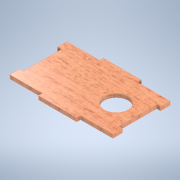
# Autodesk Inventor part: SideFemale_100wx60h
Saved by Autodesk Inventor 2022.2 (Build 262287000, 287)
## iProperties
Created: 2023-04-17
Part Number: SideFemale_100wx60h
Material: Wood (Oak)
Document SubType Name: Modeling
Designer: jaege
Density: 0.76 g/cm^3
Appearance: Red Oak - Natural Low Gloss
Author: jaege
Autodesk Inventor part; units mm, degrees
ref_plane "YZ Plane" through (0, 0, 0) normal (1, 0, 0) x (0, 1, 0)
ref_plane "XZ Plane" through (0, 0, 0) normal (0, 1, 0) x (-1, 0, 0)
ref_plane "XY Plane" through (0, 0, 0) normal (0, 0, 1) x (1, 0, 0)
sketch "Sketch1" plane through (0, 0, 0) normal (0, 1, 0) x (-1, 0, 0)
  line L0 (50, 30) -> (-50, 30) construction
  line L1 (-50, 30) -> (-50, -30) construction
  line L2 (-50, -30) -> (50, -30) construction
  line L3 (50, -30) -> (50, 30) construction
  line L4 (-50, -20) -> (-54, -20)
  line L5 (-54, -20) -> (-54, -30)
  line L6 (-54, -30) -> (-50, -30)
  line L7 (-50, -30) -> (-50, -20) construction
  line L8 (-50, 20) -> (-54, 20)
  line L9 (-54, 20) -> (-54, 30)
  line L10 (-54, 30) -> (-50, 30)
  line L11 (-50, 30) -> (-50, 20) construction
  line L12 (50, 30) -> (54, 30)
  line L13 (54, 30) -> (54, 20)
  line L14 (54, 20) -> (50, 20)
  line L15 (50, 20) -> (50, 30) construction
  line L16 (50, -30) -> (54, -30)
  line L17 (54, -30) -> (54, -20)
  line L18 (54, -20) -> (50, -20)
  line L19 (50, -20) -> (50, -30) construction
  line L20 (20, -30) -> (50, -30) construction
  line L21 (50, -30) -> (50, -34) construction
  line L22 (50, -34) -> (20, -34) construction
  line L23 (20, -34) -> (20, -30)
  line L24 (-20, -30) -> (-50, -30) construction
  line L25 (-50, -30) -> (-50, -34) construction
  line L26 (-50, -34) -> (-20, -34) construction
  line L27 (-20, -34) -> (-20, -30)
  line L28 (-50, 30) -> (-20, 30)
  line L29 (-20, 30) -> (-20, 34)
  line L30 (-20, 34) -> (-50, 34) construction
  line L31 (-50, 34) -> (-50, 30) construction
  line L32 (20, 34) -> (50, 34) construction
  line L33 (50, 34) -> (50, 30) construction
  line L34 (50, 30) -> (20, 30)
  line L35 (20, 30) -> (20, 34)
  line L36 (20, -30) -> (-20, -30) construction
  line L37 (-50, 20) -> (-50, -20)
  line L38 (50, -20) -> (50, 20)
  line L39 (20, 30) -> (-20, 30) construction
  line L40 (50, -30) -> (20, -30)
  line L41 (20, -34) -> (-20, -34)
  line L42 (-20, -30) -> (-50, -30)
  line L43 (-20, 34) -> (20, 34)
  line L44 (20, 30) -> (50, 30)
  point P0 (0, 0)
  point P1 (52, 20)
  point P2 (52, -20)
  point P3 (-20, -32)
  point P4 (20, -32)
  point P5 (0, -30)
  point P6 (50, 0)
  dimension "d0" = 100
  dimension "d1" = 60
  dimension "d2" = 4
  dimension "d3" = 40
  dimension "d4" = 40
  constraints: 90 end point, 20 parallel, 16 point on line, 12 perpendicular, 10 horizontal, 7 collinear, 6 midpoint, 5 equal length, 3 coincident, 2 horizontal alignment, 1 vertical alignment
  measures "d0" distance between parallel lines of L1 L3
  measures "d1" distance between parallel lines of L0 L2
  measures "d2" distance of L20.end L21.end
  measures "d3" distance of point (52, 20) point (52, -20)
  measures "d4" distance of point (-20, -32) point (20, -32)
extrude "Extrusion1" add sketch "Sketch1" along normal blind 4
sketch "Sketch2" plane through (0, 4, 0) normal (0, 1, 0) x (1, 0, 0)
  circle A0 centre (27.5, 0) radius 12.5
  line L0 (50, -20) -> (50, 20) projected
  point P0 (0, 0)
  dimension "d7" = 25
  dimension "d8" = 10
  constraints: 1 centre point, 1 horizontal alignment
  measures "d7" diameter of A0
  measures "d8" distance edge to line of A0 L0
extrude "Extrusion2" cut sketch "Sketch2" against normal blind 4
body "Solid1"
